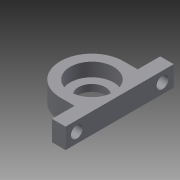
# Autodesk Inventor part: bearing_holder_plate_tb
Saved by Autodesk Inventor 2015 (Build 190159000, 159)
## iProperties
Created: 2018-01-11
Part Number: bearing_holder_plate_tb
Material: Generic
Document SubType Name: Modeling
Designer: Anshul
Density: 1 g/cm^3
Appearance: Default
Author: Anshul
Autodesk Inventor part; units mm, degrees
ref_plane "YZ Plane" through (0, 0, 0) normal (1, 0, 0) x (0, 1, 0)
ref_plane "XZ Plane" through (0, 0, 0) normal (0, 1, 0) x (-1, 0, 0)
ref_plane "XY Plane" through (0, 0, 0) normal (0, 0, 1) x (1, 0, 0)
sketch "Sketch1" plane through (0, 0, 0) normal (0, 1, 0) x (-1, 0, 0)
  line L0 (0, 0) -> (12.3, 0)
  circle A0 centre (12.3, 0) radius 9.65
  circle A1 centre (12.3, 0) radius 6
  arc A2 (12.3, -14) -> (12.3, 14) centre (12.3, 0) ccw
  line L1 (12.3, 14) -> (0, 14)
  line L2 (0, 14) -> (0, 24)
  line L3 (0, 24) -> (6, 24)
  line L4 (6, 24) -> (6, 14)
  line L5 (12.3, -14) -> (0, -14)
  line L6 (0, -14) -> (0, -24)
  line L7 (0, -24) -> (6, -24)
  line L8 (6, -24) -> (6, -14)
  line L9 (0, 14) -> (0, -14)
  dimension "d0" = 12.3
  dimension "d1" = 19.3
  dimension "d2" = 12
  dimension "d3" = 28
  dimension "d4" = 10
  dimension "d5" = 6
  dimension "d6" = 10
  constraints: 20 end point, 6 point on line, 4 perpendicular, 3 centre point, 3 coincident, 2 horizontal, 2 point on circle, 2 tangent, 1 parallel, 1 vertical
  measures "d0" distance of L0.start L0.end
  measures "d1" diameter of A0
  measures "d2" diameter of A1
  measures "d3" diameter of A2
  measures "d4" distance of L1.end L2.end
  measures "d5" distance of L2.end L3.end
  measures "d6" distance of L5.end L6.end
extrude "Extrusion1" add sketch "Sketch1" along normal blind 3 contours A0
extrude "Extrusion2" add sketch "Sketch1" along normal blind 9 contours L9 L1 A2 L5 | L2 L3 L4 L1 | L5 L8 L7 L6
sketch "Sketch2" plane through (0, 0, 24) normal (1, 0, 0) x (0, 0, -1)
  line L0 (0, 0) -> (0, 9) projected
  line L1 (0, 4.5) -> (5, 4.5)
  line L2 (48, 0) -> (48, 9) projected
  line L3 (48, 4.5) -> (43, 4.5)
  circle A0 centre (5, 4.5) radius 2.6
  circle A1 centre (43, 4.5) radius 2.6
  point P0 (24, 0)
  dimension "d11" = 5
  dimension "d12" = 5
  dimension "d13" = 5.2
  dimension "d14" = 5.2
  constraints: 4 end point, 2 centre point, 2 coincident, 2 midpoint, 1 horizontal, 1 point on line
  measures "d11" distance of L1.start L1.end
  measures "d12" distance of L3.start L3.end
  measures "d13" diameter of A0
  measures "d14" diameter of A1
extrude "Extrusion3" cut sketch "Sketch2" against normal blind 9
body "Solid1"
